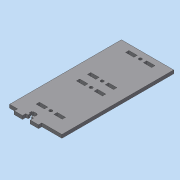
# Autodesk Inventor part: Part8
Saved by Autodesk Inventor 2016 SP1 (Build 200210100, 210)
## iProperties
Created: 2016-03-24
Part Number: Part8
Material: Generic
Document SubType Name: Modeling
Designer: Mohamed A.
Density: 1 g/cm^3
Appearance: Default
Author: Mohamed A.
Autodesk Inventor part; units mm, degrees
ref_plane "YZ Plane" through (0, 0, 0) normal (1, 0, 0) x (0, 1, 0)
ref_plane "XZ Plane" through (0, 0, 0) normal (0, 1, 0) x (-1, 0, 0)
ref_plane "XY Plane" through (0, 0, 0) normal (0, 0, 1) x (1, 0, 0)
sketch "Sketch1" plane through (0, 0, 0) normal (0, 0, 1) x (1, 0, 0)
  line L0 (19.1414, -92.5) -> (-27.8586, -92.5) construction
  line L1 (0, 3) -> (19.1414, 3) construction
  line L2 (6.5333, -102.5) -> (6.5333, -92.5) construction
  line L3 (-26.1333, -92.5) -> (-26.1333, -102.5) construction
  line L4 (-26.1333, -92.5) -> (-20.6889, -92.5)
  line L5 (19.1414, 3) -> (-27.8586, 3)
  line L6 (-27.8586, 3) -> (-27.8586, -92.5)
  line L7 (-27.8586, -92.5) -> (-20.6889, -92.5)
  line L8 (19.1414, -92.5) -> (19.1414, 3)
  line L9 (-27.8586, 3) -> (19.1414, 3)
  line L10 (19.1414, 3) -> (19.1414, 8)
  line L11 (19.1414, 8) -> (-27.8586, 8)
  line L12 (-27.8586, 8) -> (-27.8586, 3)
  line L13 (-6.3, -92.5) -> (-6.3, -95.5)
  line L14 (-6.3, -95.5) -> (1.0889, -95.5)
  line L15 (1.0889, -95.5) -> (1.0889, -92.5)
  line L16 (-13.3, -92.5) -> (-13.3, -95.5)
  line L17 (-13.3, -95.5) -> (-20.6889, -95.5)
  line L18 (-20.6889, -95.5) -> (-20.6889, -92.5)
  line L19 (-8.3, -92.5) -> (-8.3, -90.5)
  line L20 (-8.3, -90.5) -> (-7.15, -90.5)
  line L21 (-7.15, -90.5) -> (-7.15, -88.1)
  line L22 (-7.15, -88.1) -> (-8.3, -88.1)
  line L23 (-8.3, -88.1) -> (-8.3, -87.5)
  line L24 (-8.3, -87.5) -> (-11.3, -87.5)
  line L25 (-11.3, -87.5) -> (-11.3, -88.1)
  line L26 (-11.3, -88.1) -> (-12.45, -88.1)
  line L27 (-12.45, -88.1) -> (-12.45, -90.5)
  line L28 (-12.45, -90.5) -> (-11.3, -90.5)
  line L29 (-11.3, -92.5) -> (-11.3, -90.5)
  line L30 (-8.3, -92.5) -> (-6.3, -92.5)
  line L31 (-13.3, -92.5) -> (-11.3, -92.5)
  line L32 (-9.8, -83.4221) -> (-9.8, -94.6081) construction
  line L33 (-13.3, -92.5) -> (-11.3, -92.5)
  line L34 (1.0889, -92.5) -> (19.1414, -92.5)
  dimension "d4" = 5
  dimension "d13" = 5.3
  dimension "d14" = 2.4
  dimension "d15" = 3
  dimension "d16" = 32.6667
  dimension "d18" = 5.4444
  dimension "d19" = 5.4444
  dimension "d20" = 21.7778
  dimension "d21" = 7
  dimension "d22" = 3
  dimension "d23" = 5
  dimension "d24" = 8
  constraints: 62 end point, 22 perpendicular, 14 point on line, 6 parallel, 5 horizontal, 2 vertical, 4 other
  measures "d4" distance of L10.end L9.end
  measures "d13" distance between parallel lines of L27 L21
  measures "d14" distance between parallel lines of L20 L22
  measures "d15" distance between parallel lines of L29 L19
  measures "d16" distance between parallel lines of L3 L2
  measures "d18" distance between parallel lines of L2 L15
  measures "d19" distance between parallel lines of L3 L18
  measures "d20" distance between parallel lines of L18 L15
  measures "d21" distance between parallel lines of L16 L13
  measures "d22" distance between parallel lines of L14 L0
  measures "d23" distance between parallel lines of L14 L20
  measures "d24" distance between parallel lines of L14 L24
extrude "Extrusion1" add sketch "Sketch1" along normal blind 3
sketch "Sketch2" plane through (0, 0, 3) normal (0, 0, 1) x (1, 0, 0)
  line L0 (7.3914, 0) -> (-0.1086, 0) projected
  line L1 (7.3914, 0) -> (7.3914, 3) projected
  line L2 (-0.1086, 3) -> (7.3914, 3) projected
  line L3 (-0.1086, 0) -> (-0.1086, 3) projected
  line L4 (-8.6086, 0) -> (-15.7666, 0) projected
  line L5 (-8.6086, 0) -> (-8.6086, 3) projected
  line L6 (-15.7666, 3) -> (-8.6086, 3) projected
  line L7 (7.3914, -34.3) -> (-0.1086, -34.3) projected
  line L8 (7.3914, -34.3) -> (7.3914, -31.3) projected
  line L9 (-0.1086, -31.3) -> (7.3914, -31.3) projected
  line L10 (-0.1086, -34.3) -> (-0.1086, -31.3) projected
  line L11 (-8.6086, -34.3) -> (-15.7666, -34.3) projected
  line L12 (-8.6086, -34.3) -> (-8.6086, -31.3) projected
  line L13 (-15.7666, -31.3) -> (-8.6086, -31.3) projected
  line L14 (7.3914, -44.3) -> (-0.1086, -44.3) projected
  line L15 (7.3914, -44.3) -> (7.3914, -41.3) projected
  line L16 (-0.1086, -41.3) -> (7.3914, -41.3) projected
  line L17 (-0.1086, -44.3) -> (-0.1086, -41.3) projected
  line L18 (-8.6086, -44.3) -> (-15.7666, -44.3) projected
  line L19 (-8.6086, -44.3) -> (-8.6086, -41.3) projected
  line L20 (-15.7666, -41.3) -> (-8.6086, -41.3) projected
  line L21 (-0.1086, -80.5) -> (7.3914, -80.5) projected
  line L22 (7.3914, -80.5) -> (7.3914, -77.5) projected
  line L23 (-0.1086, -77.5) -> (7.3914, -77.5) projected
  line L24 (-0.1086, -80.5) -> (-0.1086, -77.5) projected
  line L25 (-15.7666, -80.5) -> (-8.6086, -80.5) projected
  line L26 (-8.6086, -80.5) -> (-8.6086, -77.5) projected
  line L27 (-15.7666, -77.5) -> (-8.6086, -77.5) projected
  line L28 (-15.7666, -80.5) -> (-15.7666, -77.5) projected
  line L29 (-0.1086, 0) -> (-8.6086, 3) construction
  line L30 (-8.6086, 0) -> (-0.1086, 3) construction
  line L31 (-8.6086, -34.3) -> (-0.1086, -31.3) construction
  line L32 (-0.1086, -34.3) -> (-8.6086, -31.3) construction
  line L33 (-8.6086, -44.3) -> (-0.1086, -41.3) construction
  line L34 (-0.1086, -44.3) -> (-8.6086, -41.3) construction
  circle A0 centre (-4.3586, 1.5) radius 1.35
  circle A1 centre (-4.3586, -32.8) radius 1.35
  circle A2 centre (-4.3586, -42.8) radius 1.35
  line L35 (-0.1086, -77.5) -> (-8.6086, -80.5) construction
  line L36 (-8.6086, -77.5) -> (-0.1086, -80.5) construction
  circle A3 centre (-4.3586, -79) radius 1.35
  line L37 (-15.7666, 0) -> (-15.7666, 3) projected
  line L38 (-15.7666, -44.3) -> (-15.7666, -41.3) projected
  line L39 (-15.7666, -34.3) -> (-15.7666, -31.3) projected
  point P0 (0, 0)
  dimension "d5" = 2.7
  dimension "d6" = 2.7
  dimension "d7" = 2.7
  dimension "d8" = 2.7
  constraints: 16 end point, 4 centre point, 4 midpoint, 4 parallel, 2 point on line
  measures "d5" diameter of A0
  measures "d6" diameter of A1
  measures "d7" diameter of A2
  measures "d8" diameter of A3
extrude "Extrusion2" cut sketch "Sketch2" against normal blind 3
equation "\"d18\" = 0.166667 * d16"
equation "\"d19\" = d18"
body "Solid1"
